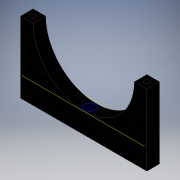
# Autodesk Inventor part: Cap_Holder_1
Saved by Autodesk Inventor 2016 (Build 200138000, 138)
## iProperties
Created: 2018-04-30
Part Number: Cap_Holder_1
Material: Generic
Document SubType Name: Modeling
Designer: Phil Erle
Density: 1 g/cm^3
Appearance: Black
Author: Phil Erle
Autodesk Inventor part; units mm, degrees
ref_plane "YZ Plane" through (0, 0, 0) normal (1, 0, 0) x (0, 1, 0)
ref_plane "XZ Plane" through (0, 0, 0) normal (0, 1, 0) x (-1, 0, 0)
ref_plane "XY Plane" through (0, 0, 0) normal (0, 0, 1) x (1, 0, 0)
sketch "Sketch1" plane through (0, 0, 0) normal (0, 0, 1) x (1, 0, 0)
  line L0 (-40, -4) -> (40, -4)
  line L1 (40, -4) -> (40, 4)
  line L2 (40, 4) -> (-40, 4)
  line L3 (-40, 4) -> (-40, -4)
  line L4 (-40, -4) -> (40, 4) construction
  line L5 (40, -4) -> (-40, 4) construction
  point P0 (0, 0)
  dimension "d0" = 80
  dimension "d1" = 8
  constraints: 12 end point, 2 midpoint, 2 parallel, 1 horizontal, 1 perpendicular
  measures "d0" distance of L2.end L1.end
  measures "d1" distance of L1.end L0.end
extrude "Extrusion1" add sketch "Sketch1" along normal blind 45
sketch "Sketch2" plane through (-40, 4, 0) normal (0, 1, 0) x (1, 0, 0)
  line L0 (80, -45) -> (0, -45) projected
  circle A0 centre (40, -45) radius 32
  point P0 (40, 0)
  dimension "d4" = 64
  constraints: 1 centre point, 1 midpoint
  measures "d4" diameter of A0
extrude "Extrusion2" cut sketch "Sketch2" against normal through all
ref_plane "Work Plane1" through (0, 0, 13.25) normal (0, 0, -1) x (-1, 0, 0)
sketch "Sketch3" plane through (0, 0, 13.25) normal (0, 0, -1) x (-1, 0, 0)
  point P0 (0, 0)
  point P1 (0, 0)
  constraints: 1 coincident
hole "Hole1" at (0, 0, 13.25) direction (0, 0, -1) diameter 3.4 end through all counterbore diameter 6.5 counterbore depth 3.4 clearance for "Socket Head Cap Screw DIN EN ISO 4762" size "M3" standard "DIN"
sketch "Sketch4" plane through (0, 0, 45) normal (0, 0, 1) x (1, 0, 0)
  line L0 (40, -4) -> (40, 4) projected
  line L1 (-40, 4) -> (-40, -4) projected
  point P0 (0, 0)
  point P1 (36, 0)
  point P2 (-36, 0)
  dimension "d15" = 4
  dimension "d16" = 4
  constraints: 2 horizontal alignment
  measures "d15" distance from line of L0 point (36, 0)
  measures "d16" distance from line of L1 point (-36, 0)
hole "Hole2" at (36, 0, 45) at (-36, 0, 45) direction (0, 0, -1) diameter 3.4 depth 12 tip angle 118 clearance for "Socket Head Cap Screw DIN EN ISO 4762" size "M3" standard "DIN"
body "Solid1"
